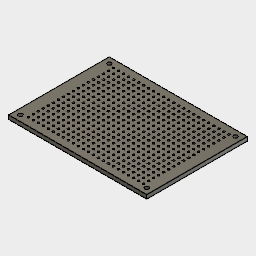
Perfboard (Autodesk Fusion 360 design; units mm, degrees)
Autodesk Fusion 360 part; units mm, degrees
sketch "Sketch3" plane through (0, 0, 0) normal (0, 1, 0) x (1, 0, 0)
  line L0 (0, 0) -> (70, 0)
  line L1 (70, 0) -> (70, 51)
  line L2 (70, 51) -> (0, 51)
  line L3 (0, 51) -> (0, 0)
  line L4 (4.5004, 2.9992) -> (65.5004, 2.9992)
  line L5 (65.5004, 2.9992) -> (65.5004, 47.9992)
  line L6 (65.5004, 47.9992) -> (4.5004, 47.9992)
  line L7 (4.5004, 47.9992) -> (4.5004, 2.9992)
  circle A0 centre (3, 3) radius 1
  circle A1 centre (3, 47.995) radius 1
  circle A2 centre (67, 3) radius 1
  circle A3 centre (67, 48) radius 1
  circle A4 centre (6, 4) radius 0.5
  circle A5 centre (6, 6.54) radius 0.5
  circle A6 centre (6, 9.08) radius 0.5
  circle A7 centre (6, 11.62) radius 0.5
  circle A8 centre (6, 21.78) radius 0.5
  circle A9 centre (6, 19.24) radius 0.5
  circle A10 centre (6, 16.7) radius 0.5
  circle A11 centre (6, 14.16) radius 0.5
  circle A12 centre (6, 24.32) radius 0.5
  circle A13 centre (6, 37.02) radius 0.5
  circle A14 centre (6, 26.86) radius 0.5
  circle A15 centre (6, 39.56) radius 0.5
  circle A16 centre (6, 29.4) radius 0.5
  circle A17 centre (6, 42.1) radius 0.5
  circle A18 centre (6, 34.48) radius 0.5
  circle A19 centre (6, 31.94) radius 0.5
  circle A20 centre (6, 44.64) radius 0.5
  circle A21 centre (6, 47.18) radius 0.5
  circle A22 centre (8.54, 6.54) radius 0.5
  circle A23 centre (8.54, 14.16) radius 0.5
  circle A24 centre (8.54, 24.32) radius 0.5
  circle A25 centre (8.54, 31.94) radius 0.5
  circle A26 centre (8.54, 26.86) radius 0.5
  circle A27 centre (8.54, 42.1) radius 0.5
  circle A28 centre (8.54, 34.48) radius 0.5
  circle A29 centre (8.54, 29.4) radius 0.5
  circle A30 centre (8.54, 16.7) radius 0.5
  circle A31 centre (8.54, 37.02) radius 0.5
  circle A32 centre (8.54, 21.78) radius 0.5
  circle A33 centre (8.54, 44.64) radius 0.5
  circle A34 centre (8.54, 19.24) radius 0.5
  circle A35 centre (8.54, 11.62) radius 0.5
  circle A36 centre (8.54, 4) radius 0.5
  circle A37 centre (8.54, 9.08) radius 0.5
  circle A38 centre (8.54, 39.56) radius 0.5
  circle A39 centre (8.54, 47.18) radius 0.5
  circle A40 centre (11.08, 34.48) radius 0.5
  circle A41 centre (13.62, 31.94) radius 0.5
  circle A42 centre (13.62, 19.24) radius 0.5
  circle A43 centre (11.08, 6.54) radius 0.5
  circle A44 centre (11.08, 21.78) radius 0.5
  circle A45 centre (11.08, 16.7) radius 0.5
  circle A46 centre (11.08, 14.16) radius 0.5
  circle A47 centre (11.08, 24.32) radius 0.5
  circle A48 centre (13.62, 44.64) radius 0.5
  circle A49 centre (13.62, 37.02) radius 0.5
  circle A50 centre (13.62, 16.7) radius 0.5
  circle A51 centre (13.62, 29.4) radius 0.5
  circle A52 centre (11.08, 9.08) radius 0.5
  circle A53 centre (11.08, 42.1) radius 0.5
  circle A54 centre (11.08, 26.86) radius 0.5
  circle A55 centre (13.62, 11.62) radius 0.5
  circle A56 centre (13.62, 34.48) radius 0.5
  circle A57 centre (13.62, 26.86) radius 0.5
  circle A58 centre (13.62, 6.54) radius 0.5
  circle A59 centre (13.62, 24.32) radius 0.5
  circle A60 centre (11.08, 47.18) radius 0.5
  circle A61 centre (13.62, 21.78) radius 0.5
  circle A62 centre (13.62, 42.1) radius 0.5
  circle A63 centre (11.08, 19.24) radius 0.5
  circle A64 centre (11.08, 31.94) radius 0.5
  circle A65 centre (11.08, 44.64) radius 0.5
  circle A66 centre (11.08, 4) radius 0.5
  circle A67 centre (11.08, 11.62) radius 0.5
  circle A68 centre (11.08, 37.02) radius 0.5
  circle A69 centre (11.08, 39.56) radius 0.5
  circle A70 centre (11.08, 29.4) radius 0.5
  circle A71 centre (13.62, 14.16) radius 0.5
  circle A72 centre (13.62, 39.56) radius 0.5
  circle A73 centre (13.62, 9.08) radius 0.5
  circle A74 centre (13.62, 47.18) radius 0.5
  circle A75 centre (13.62, 4) radius 0.5
  circle A76 centre (21.24, 24.32) radius 0.5
  circle A77 centre (21.24, 14.16) radius 0.5
  circle A78 centre (23.78, 6.54) radius 0.5
  circle A79 centre (21.24, 42.1) radius 0.5
  circle A80 centre (23.78, 44.64) radius 0.5
  circle A81 centre (18.7, 47.18) radius 0.5
  circle A82 centre (23.78, 34.48) radius 0.5
  circle A83 centre (23.78, 29.4) radius 0.5
  circle A84 centre (23.78, 16.7) radius 0.5
  circle A85 centre (23.78, 24.32) radius 0.5
  circle A86 centre (23.78, 26.86) radius 0.5
  circle A87 centre (21.24, 26.86) radius 0.5
  circle A88 centre (23.78, 11.62) radius 0.5
  circle A89 centre (21.24, 9.08) radius 0.5
  circle A90 centre (23.78, 37.02) radius 0.5
  circle A91 centre (23.78, 19.24) radius 0.5
  circle A92 centre (23.78, 31.94) radius 0.5
  circle A93 centre (18.7, 34.48) radius 0.5
  circle A94 centre (21.24, 34.48) radius 0.5
  circle A95 centre (16.16, 14.16) radius 0.5
  circle A96 centre (16.16, 44.64) radius 0.5
  circle A97 centre (16.16, 47.18) radius 0.5
  circle A98 centre (16.16, 34.48) radius 0.5
  circle A99 centre (16.16, 26.86) radius 0.5
  circle A100 centre (16.16, 9.08) radius 0.5
  circle A101 centre (16.16, 39.56) radius 0.5
  circle A102 centre (16.16, 31.94) radius 0.5
  circle A103 centre (16.16, 16.7) radius 0.5
  circle A104 centre (16.16, 11.62) radius 0.5
  circle A105 centre (16.16, 37.02) radius 0.5
  circle A106 centre (16.16, 19.24) radius 0.5
  circle A107 centre (16.16, 29.4) radius 0.5
  circle A108 centre (18.7, 6.54) radius 0.5
  circle A109 centre (18.7, 14.16) radius 0.5
  circle A110 centre (18.7, 24.32) radius 0.5
  circle A111 centre (16.16, 4) radius 0.5
  circle A112 centre (16.16, 21.78) radius 0.5
  circle A113 centre (18.7, 31.94) radius 0.5
  circle A114 centre (16.16, 24.32) radius 0.5
  circle A115 centre (18.7, 26.86) radius 0.5
  circle A116 centre (16.16, 42.1) radius 0.5
  circle A117 centre (18.7, 42.1) radius 0.5
  circle A118 centre (16.16, 6.54) radius 0.5
  circle A119 centre (21.24, 6.54) radius 0.5
  circle A120 centre (21.24, 16.7) radius 0.5
  circle A121 centre (18.7, 9.08) radius 0.5
  circle A122 centre (21.24, 21.78) radius 0.5
  circle A123 centre (18.7, 11.62) radius 0.5
  circle A124 centre (23.78, 39.56) radius 0.5
  circle A125 centre (21.24, 44.64) radius 0.5
  circle A126 centre (21.24, 31.94) radius 0.5
  circle A127 centre (21.24, 11.62) radius 0.5
  circle A128 centre (18.7, 37.02) radius 0.5
  circle A129 centre (21.24, 39.56) radius 0.5
  circle A130 centre (23.78, 42.1) radius 0.5
  circle A131 centre (18.7, 21.78) radius 0.5
  circle A132 centre (23.78, 21.78) radius 0.5
  circle A133 centre (23.78, 9.08) radius 0.5
  circle A134 centre (23.78, 14.16) radius 0.5
  circle A135 centre (21.24, 47.18) radius 0.5
  circle A136 centre (21.24, 19.24) radius 0.5
  circle A137 centre (18.7, 4) radius 0.5
  circle A138 centre (21.24, 4) radius 0.5
  circle A139 centre (18.7, 29.4) radius 0.5
  circle A140 centre (18.7, 44.64) radius 0.5
  circle A141 centre (21.24, 37.02) radius 0.5
  circle A142 centre (18.7, 16.7) radius 0.5
  circle A143 centre (23.78, 4) radius 0.5
  circle A144 centre (18.7, 19.24) radius 0.5
  circle A145 centre (21.24, 29.4) radius 0.5
  circle A146 centre (23.78, 47.18) radius 0.5
  circle A147 centre (18.7, 39.56) radius 0.5
  circle A148 centre (39.02, 42.1) radius 0.5
  circle A149 centre (36.48, 37.02) radius 0.5
  circle A150 centre (36.48, 11.62) radius 0.5
  circle A151 centre (41.56, 34.48) radius 0.5
  circle A152 centre (39.02, 6.54) radius 0.5
  circle A153 centre (36.48, 42.1) radius 0.5
  circle A154 centre (36.48, 19.24) radius 0.5
  circle A155 centre (36.48, 4) radius 0.5
  circle A156 centre (39.02, 26.86) radius 0.5
  circle A157 centre (36.48, 24.32) radius 0.5
  circle A158 centre (36.48, 29.4) radius 0.5
  circle A159 centre (39.02, 31.94) radius 0.5
  circle A160 centre (36.48, 21.78) radius 0.5
  circle A161 centre (39.02, 24.32) radius 0.5
  circle A162 centre (39.02, 14.16) radius 0.5
  circle A163 centre (36.48, 39.56) radius 0.5
  circle A164 centre (36.48, 9.08) radius 0.5
  circle A165 centre (31.4, 47.18) radius 0.5
  circle A166 centre (33.94, 6.54) radius 0.5
  circle A167 centre (33.94, 42.1) radius 0.5
  circle A168 centre (31.4, 31.94) radius 0.5
  circle A169 centre (31.4, 37.02) radius 0.5
  circle A170 centre (31.4, 39.56) radius 0.5
  circle A171 centre (33.94, 9.08) radius 0.5
  circle A172 centre (33.94, 47.18) radius 0.5
  circle A173 centre (33.94, 34.48) radius 0.5
  circle A174 centre (33.94, 14.16) radius 0.5
  circle A175 centre (33.94, 4) radius 0.5
  circle A176 centre (39.02, 39.56) radius 0.5
  circle A177 centre (44.1, 47.18) radius 0.5
  circle A178 centre (41.56, 29.4) radius 0.5
  circle A179 centre (33.94, 21.78) radius 0.5
  circle A180 centre (44.1, 4) radius 0.5
  circle A181 centre (39.02, 19.24) radius 0.5
  circle A182 centre (33.94, 39.56) radius 0.5
  circle A183 centre (39.02, 16.7) radius 0.5
  circle A184 centre (33.94, 24.32) radius 0.5
  circle A185 centre (41.56, 37.02) radius 0.5
  circle A186 centre (39.02, 34.48) radius 0.5
  circle A187 centre (31.4, 19.24) radius 0.5
  circle A188 centre (31.4, 29.4) radius 0.5
  circle A189 centre (33.94, 26.86) radius 0.5
  circle A190 centre (31.4, 4) radius 0.5
  circle A191 centre (31.4, 11.62) radius 0.5
  circle A192 centre (31.4, 44.64) radius 0.5
  circle A193 centre (36.48, 14.16) radius 0.5
  circle A194 centre (36.48, 16.7) radius 0.5
  circle A195 centre (36.48, 47.18) radius 0.5
  circle A196 centre (36.48, 31.94) radius 0.5
  circle A197 centre (28.86, 34.48) radius 0.5
  circle A198 centre (28.86, 42.1) radius 0.5
  circle A199 centre (31.4, 42.1) radius 0.5
  circle A200 centre (31.4, 26.86) radius 0.5
  circle A201 centre (28.86, 47.18) radius 0.5
  circle A202 centre (28.86, 37.02) radius 0.5
  circle A203 centre (28.86, 44.64) radius 0.5
  circle A204 centre (33.94, 31.94) radius 0.5
  circle A205 centre (33.94, 16.7) radius 0.5
  circle A206 centre (33.94, 11.62) radius 0.5
  circle A207 centre (31.4, 14.16) radius 0.5
  circle A208 centre (28.86, 39.56) radius 0.5
  circle A209 centre (28.86, 9.08) radius 0.5
  circle A210 centre (28.86, 4) radius 0.5
  circle A211 centre (31.4, 6.54) radius 0.5
  circle A212 centre (33.94, 37.02) radius 0.5
  circle A213 centre (28.86, 21.78) radius 0.5
  circle A214 centre (33.94, 29.4) radius 0.5
  circle A215 centre (28.86, 11.62) radius 0.5
  circle A216 centre (31.4, 34.48) radius 0.5
  circle A217 centre (28.86, 29.4) radius 0.5
  circle A218 centre (31.4, 16.7) radius 0.5
  circle A219 centre (31.4, 24.32) radius 0.5
  circle A220 centre (28.86, 16.7) radius 0.5
  circle A221 centre (33.94, 44.64) radius 0.5
  circle A222 centre (31.4, 9.08) radius 0.5
  circle A223 centre (28.86, 19.24) radius 0.5
  circle A224 centre (33.94, 19.24) radius 0.5
  circle A225 centre (31.4, 21.78) radius 0.5
  circle A226 centre (36.48, 44.64) radius 0.5
  circle A227 centre (26.32, 29.4) radius 0.5
  circle A228 centre (26.32, 4) radius 0.5
  circle A229 centre (26.32, 42.1) radius 0.5
  circle A230 centre (26.32, 21.78) radius 0.5
  circle A231 centre (26.32, 34.48) radius 0.5
  circle A232 centre (26.32, 31.94) radius 0.5
  circle A233 centre (26.32, 47.18) radius 0.5
  circle A234 centre (28.86, 6.54) radius 0.5
  circle A235 centre (26.32, 44.64) radius 0.5
  circle A236 centre (28.86, 14.16) radius 0.5
  circle A237 centre (26.32, 26.86) radius 0.5
  circle A238 centre (28.86, 24.32) radius 0.5
  circle A239 centre (26.32, 9.08) radius 0.5
  circle A240 centre (26.32, 14.16) radius 0.5
  circle A241 centre (26.32, 37.02) radius 0.5
  circle A242 centre (26.32, 39.56) radius 0.5
  circle A243 centre (26.32, 24.32) radius 0.5
  circle A244 centre (26.32, 6.54) radius 0.5
  circle A245 centre (26.32, 16.7) radius 0.5
  circle A246 centre (26.32, 11.62) radius 0.5
  circle A247 centre (26.32, 19.24) radius 0.5
  circle A248 centre (28.86, 31.94) radius 0.5
  circle A249 centre (28.86, 26.86) radius 0.5
  circle A250 centre (36.48, 26.86) radius 0.5
  circle A251 centre (41.56, 4) radius 0.5
  circle A252 centre (39.02, 4) radius 0.5
  circle A253 centre (39.02, 37.02) radius 0.5
  circle A254 centre (41.56, 44.64) radius 0.5
  circle A255 centre (44.1, 39.56) radius 0.5
  circle A256 centre (39.02, 11.62) radius 0.5
  circle A257 centre (39.02, 9.08) radius 0.5
  circle A258 centre (41.56, 6.54) radius 0.5
  circle A259 centre (36.48, 6.54) radius 0.5
  circle A260 centre (39.02, 21.78) radius 0.5
  circle A261 centre (41.56, 21.78) radius 0.5
  circle A262 centre (44.1, 14.16) radius 0.5
  circle A263 centre (41.56, 16.7) radius 0.5
  circle A264 centre (36.48, 34.48) radius 0.5
  circle A265 centre (41.56, 11.62) radius 0.5
  circle A266 centre (44.1, 9.08) radius 0.5
  circle A267 centre (39.02, 44.64) radius 0.5
  circle A268 centre (41.56, 19.24) radius 0.5
  circle A269 centre (41.56, 47.18) radius 0.5
  circle A270 centre (41.56, 39.56) radius 0.5
  circle A271 centre (44.1, 21.78) radius 0.5
  circle A272 centre (44.1, 42.1) radius 0.5
  circle A273 centre (41.56, 31.94) radius 0.5
  circle A274 centre (39.02, 29.4) radius 0.5
  circle A275 centre (44.1, 31.94) radius 0.5
  circle A276 centre (41.56, 26.86) radius 0.5
  circle A277 centre (39.02, 47.18) radius 0.5
  circle A278 centre (44.1, 19.24) radius 0.5
  circle A279 centre (41.56, 24.32) radius 0.5
  circle A280 centre (44.1, 26.86) radius 0.5
  circle A281 centre (44.1, 37.02) radius 0.5
  circle A282 centre (44.1, 44.64) radius 0.5
  circle A283 centre (44.1, 6.54) radius 0.5
  circle A284 centre (44.1, 24.32) radius 0.5
  circle A285 centre (44.1, 34.48) radius 0.5
  circle A286 centre (41.56, 14.16) radius 0.5
  circle A287 centre (41.56, 9.08) radius 0.5
  circle A288 centre (44.1, 16.7) radius 0.5
  circle A289 centre (44.1, 11.62) radius 0.5
  circle A290 centre (41.56, 42.1) radius 0.5
  circle A291 centre (44.1, 29.4) radius 0.5
  circle A292 centre (59.34, 47.18) radius 0.5
  circle A293 centre (56.8, 34.48) radius 0.5
  circle A294 centre (49.18, 29.4) radius 0.5
  circle A295 centre (49.18, 14.16) radius 0.5
  circle A296 centre (51.72, 4) radius 0.5
  circle A297 centre (54.26, 39.56) radius 0.5
  circle A298 centre (54.26, 42.1) radius 0.5
  circle A299 centre (49.18, 34.48) radius 0.5
  circle A300 centre (51.72, 21.78) radius 0.5
  circle A301 centre (46.64, 11.62) radius 0.5
  circle A302 centre (51.72, 16.7) radius 0.5
  circle A303 centre (54.26, 24.32) radius 0.5
  circle A304 centre (54.26, 14.16) radius 0.5
  circle A305 centre (46.64, 44.64) radius 0.5
  circle A306 centre (51.72, 47.18) radius 0.5
  circle A307 centre (46.64, 42.1) radius 0.5
  circle A308 centre (49.18, 44.64) radius 0.5
  circle A309 centre (46.64, 9.08) radius 0.5
  circle A310 centre (49.18, 19.24) radius 0.5
  circle A311 centre (46.64, 31.94) radius 0.5
  circle A312 centre (46.64, 39.56) radius 0.5
  circle A313 centre (49.18, 9.08) radius 0.5
  circle A314 centre (56.8, 29.4) radius 0.5
  circle A315 centre (59.34, 4) radius 0.5
  circle A316 centre (51.72, 42.1) radius 0.5
  circle A317 centre (54.26, 19.24) radius 0.5
  circle A318 centre (54.26, 16.7) radius 0.5
  circle A319 centre (49.18, 47.18) radius 0.5
  circle A320 centre (54.26, 34.48) radius 0.5
  circle A321 centre (49.18, 21.78) radius 0.5
  circle A322 centre (49.18, 31.94) radius 0.5
  circle A323 centre (51.72, 24.32) radius 0.5
  circle A324 centre (49.18, 24.32) radius 0.5
  circle A325 centre (49.18, 4) radius 0.5
  circle A326 centre (51.72, 29.4) radius 0.5
  circle A327 centre (46.64, 26.86) radius 0.5
  circle A328 centre (54.26, 6.54) radius 0.5
  circle A329 centre (51.72, 31.94) radius 0.5
  circle A330 centre (49.18, 11.62) radius 0.5
  circle A331 centre (54.26, 31.94) radius 0.5
  circle A332 centre (51.72, 14.16) radius 0.5
  circle A333 centre (46.64, 14.16) radius 0.5
  circle A334 centre (51.72, 37.02) radius 0.5
  circle A335 centre (54.26, 26.86) radius 0.5
  circle A336 centre (46.64, 19.24) radius 0.5
  circle A337 centre (51.72, 9.08) radius 0.5
  circle A338 centre (46.64, 37.02) radius 0.5
  circle A339 centre (51.72, 11.62) radius 0.5
  circle A340 centre (49.18, 39.56) radius 0.5
  circle A341 centre (49.18, 26.86) radius 0.5
  circle A342 centre (46.64, 4) radius 0.5
  circle A343 centre (46.64, 6.54) radius 0.5
  circle A344 centre (46.64, 47.18) radius 0.5
  circle A345 centre (49.18, 42.1) radius 0.5
  circle A346 centre (56.8, 37.02) radius 0.5
  circle A347 centre (49.18, 16.7) radius 0.5
  circle A348 centre (49.18, 37.02) radius 0.5
  circle A349 centre (46.64, 34.48) radius 0.5
  circle A350 centre (46.64, 16.7) radius 0.5
  circle A351 centre (49.18, 6.54) radius 0.5
  circle A352 centre (46.64, 24.32) radius 0.5
  circle A353 centre (51.72, 39.56) radius 0.5
  circle A354 centre (51.72, 19.24) radius 0.5
  circle A355 centre (46.64, 29.4) radius 0.5
  circle A356 centre (59.34, 6.54) radius 0.5
  circle A357 centre (59.34, 21.78) radius 0.5
  circle A358 centre (56.8, 31.94) radius 0.5
  circle A359 centre (56.8, 21.78) radius 0.5
  circle A360 centre (59.34, 9.08) radius 0.5
  circle A361 centre (56.8, 14.16) radius 0.5
  circle A362 centre (56.8, 4) radius 0.5
  circle A363 centre (59.34, 29.4) radius 0.5
  circle A364 centre (56.8, 47.18) radius 0.5
  circle A365 centre (56.8, 16.7) radius 0.5
  circle A366 centre (56.8, 11.62) radius 0.5
  circle A367 centre (54.26, 9.08) radius 0.5
  circle A368 centre (51.72, 26.86) radius 0.5
  circle A369 centre (59.34, 42.1) radius 0.5
  circle A370 centre (56.8, 39.56) radius 0.5
  circle A371 centre (59.34, 31.94) radius 0.5
  circle A372 centre (56.8, 6.54) radius 0.5
  circle A373 centre (56.8, 44.64) radius 0.5
  circle A374 centre (56.8, 19.24) radius 0.5
  circle A375 centre (59.34, 11.62) radius 0.5
  circle A376 centre (59.34, 39.56) radius 0.5
  circle A377 centre (59.34, 14.16) radius 0.5
  circle A378 centre (51.72, 34.48) radius 0.5
  circle A379 centre (56.8, 26.86) radius 0.5
  circle A380 centre (51.72, 6.54) radius 0.5
  circle A381 centre (54.26, 21.78) radius 0.5
  circle A382 centre (59.34, 37.02) radius 0.5
  circle A383 centre (59.34, 44.64) radius 0.5
  circle A384 centre (59.34, 24.32) radius 0.5
  circle A385 centre (54.26, 11.62) radius 0.5
  circle A386 centre (59.34, 34.48) radius 0.5
  circle A387 centre (56.8, 9.08) radius 0.5
  circle A388 centre (51.72, 44.64) radius 0.5
  circle A389 centre (54.26, 47.18) radius 0.5
  circle A390 centre (59.34, 16.7) radius 0.5
  circle A391 centre (54.26, 4) radius 0.5
  circle A392 centre (54.26, 29.4) radius 0.5
  circle A393 centre (56.8, 24.32) radius 0.5
  circle A394 centre (46.64, 21.78) radius 0.5
  circle A395 centre (56.8, 42.1) radius 0.5
  circle A396 centre (59.34, 19.24) radius 0.5
  circle A397 centre (59.34, 26.86) radius 0.5
  circle A398 centre (54.26, 44.64) radius 0.5
  circle A399 centre (54.26, 37.02) radius 0.5
  circle A400 centre (61.88, 37.02) radius 0.5
  circle A401 centre (61.88, 19.24) radius 0.5
  circle A402 centre (64.42, 47.18) radius 0.5
  circle A403 centre (64.42, 42.1) radius 0.5
  circle A404 centre (61.88, 11.62) radius 0.5
  circle A405 centre (61.88, 39.56) radius 0.5
  circle A406 centre (64.42, 39.56) radius 0.5
  circle A407 centre (61.88, 16.7) radius 0.5
  circle A408 centre (61.88, 29.4) radius 0.5
  circle A409 centre (64.42, 11.62) radius 0.5
  circle A410 centre (61.88, 34.48) radius 0.5
  circle A411 centre (61.88, 47.18) radius 0.5
  circle A412 centre (64.42, 29.4) radius 0.5
  circle A413 centre (64.42, 9.08) radius 0.5
  circle A414 centre (61.88, 14.16) radius 0.5
  circle A415 centre (61.88, 21.78) radius 0.5
  circle A416 centre (64.42, 4) radius 0.5
  circle A417 centre (64.42, 21.78) radius 0.5
  circle A418 centre (61.88, 6.54) radius 0.5
  circle A419 centre (64.42, 31.94) radius 0.5
  circle A420 centre (61.88, 44.64) radius 0.5
  circle A421 centre (61.88, 31.94) radius 0.5
  circle A422 centre (61.88, 4) radius 0.5
  circle A423 centre (64.42, 6.54) radius 0.5
  circle A424 centre (61.88, 9.08) radius 0.5
  circle A425 centre (64.42, 24.32) radius 0.5
  circle A426 centre (64.42, 44.64) radius 0.5
  circle A427 centre (64.42, 19.24) radius 0.5
  circle A428 centre (61.88, 42.1) radius 0.5
  circle A429 centre (64.42, 16.7) radius 0.5
  circle A430 centre (64.42, 34.48) radius 0.5
  circle A431 centre (61.88, 24.32) radius 0.5
  circle A432 centre (64.42, 26.86) radius 0.5
  circle A433 centre (64.42, 14.16) radius 0.5
  circle A434 centre (61.88, 26.86) radius 0.5
  circle A435 centre (64.42, 37.02) radius 0.5
  dimension "d8" = 70
  dimension "d9" = 51
  dimension "d10" = 61
  dimension "d11" = 45
  dimension "d16" = 2
  dimension "d17" = 2
  dimension "d18" = 2
  dimension "d23" = 1
  dimension "d24" = 1
  dimension "d26" = 1
  dimension "d27" = 1
  dimension "d28" = 1
  dimension "d29" = 1
  dimension "d30" = 1
  dimension "d31" = 1
  dimension "d32" = 1
  dimension "d33" = 1
  dimension "d34" = 1
  dimension "d35" = 1
  dimension "d36" = 1
  dimension "d37" = 1
  dimension "d38" = 1
  dimension "d39" = 1
  dimension "d40" = 1
  dimension "d41" = 1
  dimension "d42" = 1
  dimension "d43" = 1
  dimension "d44" = 1
  dimension "d45" = 1
  dimension "d46" = 1
  dimension "d47" = 1
  dimension "d48" = 1
  dimension "d49" = 1
  dimension "d50" = 1
  dimension "d51" = 1
  dimension "d52" = 1
  dimension "d53" = 1
  dimension "d54" = 1
  dimension "d55" = 1
  dimension "d56" = 1
  dimension "d57" = 1
  dimension "d58" = 1
  dimension "d59" = 1
  dimension "d60" = 1
  dimension "d61" = 1
  dimension "d62" = 1
  dimension "d63" = 1
  dimension "d64" = 1
  dimension "d65" = 1
  dimension "d66" = 1
  dimension "d67" = 1
  dimension "d68" = 1
  dimension "d69" = 1
  dimension "d70" = 1
  dimension "d71" = 1
  dimension "d72" = 1
  dimension "d73" = 1
  dimension "d74" = 1
  dimension "d75" = 1
  dimension "d76" = 1
  dimension "d77" = 1
  dimension "d78" = 1
  dimension "d79" = 1
  dimension "d80" = 1
  dimension "d81" = 1
  dimension "d82" = 1
  dimension "d83" = 1
  dimension "d84" = 1
  dimension "d85" = 1
  dimension "d86" = 1
  dimension "d87" = 1
  dimension "d88" = 1
  dimension "d89" = 1
  dimension "d90" = 1
  dimension "d91" = 1
  dimension "d92" = 1
  dimension "d93" = 1
  dimension "d94" = 1
  dimension "d95" = 1
  dimension "d96" = 1
  dimension "d97" = 1
  dimension "d98" = 1
  dimension "d99" = 1
  dimension "d100" = 1
  dimension "d101" = 1
  dimension "d102" = 1
  dimension "d103" = 1
  dimension "d104" = 1
  dimension "d105" = 1
  dimension "d106" = 1
  dimension "d107" = 1
  dimension "d108" = 1
  dimension "d109" = 1
  dimension "d110" = 1
  dimension "d111" = 1
  dimension "d112" = 1
  dimension "d113" = 1
  dimension "d114" = 1
  dimension "d115" = 1
  dimension "d116" = 1
  dimension "d117" = 1
  dimension "d118" = 1
  dimension "d119" = 1
  dimension "d120" = 1
  dimension "d121" = 1
  dimension "d122" = 1
  dimension "d123" = 1
  dimension "d124" = 1
  dimension "d125" = 1
  dimension "d126" = 1
  dimension "d127" = 1
  dimension "d128" = 1
  dimension "d129" = 1
  dimension "d130" = 1
  dimension "d131" = 1
  dimension "d132" = 1
  dimension "d133" = 1
  dimension "d134" = 1
  dimension "d135" = 1
  dimension "d136" = 1
  dimension "d137" = 1
  dimension "d138" = 1
  dimension "d139" = 1
  dimension "d140" = 1
  dimension "d141" = 1
  dimension "d142" = 1
  dimension "d143" = 1
  dimension "d144" = 1
  dimension "d145" = 1
  dimension "d146" = 1
  dimension "d147" = 1
  dimension "d148" = 1
  dimension "d149" = 1
  dimension "d150" = 1
  dimension "d151" = 1
  dimension "d152" = 1
  dimension "d153" = 1
  dimension "d154" = 1
  dimension "d155" = 1
  dimension "d156" = 1
  dimension "d157" = 1
  dimension "d158" = 1
  dimension "d159" = 1
  dimension "d160" = 1
  dimension "d161" = 1
  dimension "d162" = 1
  dimension "d163" = 1
  dimension "d164" = 1
  dimension "d165" = 1
  dimension "d166" = 1
  dimension "d167" = 1
  dimension "d168" = 1
  dimension "d169" = 1
  dimension "d170" = 1
  dimension "d171" = 1
  dimension "d172" = 1
  dimension "d173" = 1
  dimension "d174" = 1
  dimension "d175" = 1
  dimension "d176" = 1
  dimension "d177" = 1
  dimension "d178" = 1
  dimension "d179" = 1
  dimension "d180" = 1
  dimension "d181" = 1
  dimension "d182" = 1
  dimension "d183" = 1
  dimension "d184" = 1
  dimension "d185" = 1
  dimension "d186" = 1
  dimension "d187" = 1
  dimension "d188" = 1
  dimension "d189" = 1
  dimension "d190" = 1
  dimension "d191" = 1
  dimension "d192" = 1
  dimension "d193" = 1
  dimension "d194" = 1
  dimension "d195" = 1
  dimension "d196" = 1
  dimension "d197" = 1
  dimension "d198" = 1
  dimension "d199" = 1
  dimension "d200" = 1
  dimension "d201" = 1
  dimension "d202" = 1
  dimension "d203" = 1
  dimension "d204" = 1
  dimension "d205" = 1
  dimension "d206" = 1
  dimension "d207" = 1
  dimension "d208" = 1
  dimension "d209" = 1
  dimension "d210" = 1
  dimension "d211" = 1
  dimension "d212" = 1
  dimension "d213" = 1
  dimension "d214" = 1
  dimension "d215" = 1
  dimension "d216" = 1
  dimension "d217" = 1
  dimension "d218" = 1
  dimension "d219" = 1
  dimension "d220" = 1
  dimension "d221" = 1
  dimension "d222" = 1
  dimension "d223" = 1
  dimension "d224" = 1
  dimension "d225" = 1
  dimension "d226" = 1
  dimension "d227" = 1
  dimension "d228" = 1
  dimension "d229" = 1
  dimension "d230" = 1
  dimension "d231" = 1
  dimension "d232" = 1
  dimension "d233" = 1
  dimension "d234" = 1
  dimension "d235" = 1
  dimension "d236" = 1
  dimension "d237" = 1
  dimension "d238" = 1
  dimension "d239" = 1
  dimension "d240" = 1
  dimension "d241" = 1
  dimension "d242" = 1
  dimension "d243" = 1
  dimension "d244" = 1
  dimension "d245" = 1
  dimension "d246" = 1
  dimension "d247" = 1
  dimension "d248" = 1
  dimension "d249" = 1
  dimension "d250" = 1
  dimension "d251" = 1
  dimension "d252" = 1
  dimension "d253" = 1
  dimension "d254" = 1
  dimension "d255" = 1
  dimension "d256" = 1
  dimension "d257" = 1
  dimension "d258" = 1
  dimension "d259" = 1
  dimension "d260" = 1
  dimension "d261" = 1
  dimension "d262" = 1
  dimension "d263" = 1
  dimension "d264" = 1
  dimension "d265" = 1
  dimension "d266" = 1
  dimension "d267" = 1
  dimension "d268" = 1
  dimension "d269" = 1
  dimension "d270" = 1
  dimension "d271" = 1
  dimension "d272" = 1
  dimension "d273" = 1
  dimension "d274" = 1
  dimension "d275" = 1
  dimension "d276" = 1
  dimension "d277" = 1
  dimension "d278" = 1
  dimension "d279" = 1
  dimension "d280" = 1
  dimension "d281" = 1
  dimension "d282" = 1
  dimension "d283" = 1
  dimension "d284" = 1
  dimension "d285" = 1
  dimension "d286" = 1
  dimension "d287" = 1
  dimension "d288" = 1
  dimension "d289" = 1
  dimension "d290" = 1
  dimension "d291" = 1
  dimension "d292" = 1
  dimension "d293" = 1
  dimension "d294" = 1
  dimension "d295" = 1
  dimension "d296" = 1
  dimension "d297" = 1
  dimension "d298" = 1
  dimension "d299" = 1
  dimension "d300" = 1
  dimension "d301" = 1
  dimension "d302" = 1
  dimension "d303" = 1
  dimension "d304" = 1
  dimension "d305" = 1
  dimension "d306" = 1
  dimension "d307" = 1
  dimension "d308" = 1
  dimension "d309" = 1
  dimension "d310" = 1
  dimension "d311" = 1
  dimension "d312" = 1
  dimension "d313" = 1
  dimension "d314" = 1
  dimension "d315" = 1
  dimension "d316" = 1
  dimension "d317" = 1
  dimension "d318" = 1
  dimension "d319" = 1
  dimension "d320" = 1
  dimension "d321" = 1
  dimension "d322" = 1
  dimension "d323" = 1
  dimension "d324" = 1
  dimension "d325" = 1
  dimension "d326" = 1
  dimension "d327" = 1
  dimension "d328" = 1
  dimension "d329" = 1
  dimension "d330" = 1
  dimension "d331" = 1
  dimension "d332" = 1
  dimension "d333" = 1
  dimension "d334" = 1
  dimension "d335" = 1
  dimension "d336" = 1
  dimension "d337" = 1
  dimension "d338" = 1
  dimension "d339" = 1
  dimension "d340" = 1
  dimension "d341" = 1
  dimension "d342" = 1
  dimension "d343" = 1
  dimension "d344" = 1
  dimension "d345" = 1
  dimension "d346" = 1
  dimension "d347" = 1
  dimension "d348" = 1
  dimension "d349" = 1
  dimension "d350" = 1
  dimension "d351" = 1
  dimension "d352" = 1
  dimension "d353" = 1
  dimension "d354" = 1
  dimension "d355" = 1
  dimension "d356" = 1
  dimension "d357" = 1
  dimension "d358" = 1
  dimension "d359" = 1
  dimension "d360" = 1
  dimension "d361" = 1
  dimension "d362" = 1
  dimension "d363" = 1
  dimension "d364" = 1
  dimension "d365" = 1
  dimension "d366" = 1
  dimension "d367" = 1
  dimension "d368" = 1
  dimension "d369" = 1
  dimension "d370" = 1
  dimension "d371" = 1
  dimension "d372" = 1
  dimension "d373" = 1
  dimension "d374" = 1
  dimension "d375" = 1
  dimension "d376" = 1
  dimension "d377" = 1
  dimension "d378" = 1
  dimension "d379" = 1
  dimension "d380" = 1
  dimension "d381" = 1
  dimension "d382" = 1
  dimension "d383" = 1
  dimension "d384" = 1
  dimension "d385" = 1
  dimension "d386" = 1
  dimension "d387" = 1
  dimension "d388" = 1
  dimension "d389" = 1
  dimension "d390" = 1
  dimension "d391" = 1
  dimension "d392" = 1
  dimension "d393" = 1
  dimension "d394" = 1
  dimension "d395" = 1
  dimension "d396" = 1
  dimension "d397" = 1
  dimension "d398" = 1
  dimension "d399" = 1
  dimension "d400" = 1
  dimension "d401" = 1
  dimension "d402" = 1
  dimension "d403" = 1
  dimension "d404" = 1
  dimension "d405" = 1
  dimension "d406" = 1
  dimension "d407" = 1
  dimension "d408" = 1
  dimension "d409" = 1
  dimension "d410" = 1
  dimension "d411" = 1
  dimension "d412" = 1
  dimension "d413" = 1
  dimension "d414" = 1
  dimension "d415" = 1
  dimension "d416" = 1
  dimension "d417" = 1
  dimension "d418" = 1
  dimension "d419" = 1
  dimension "d420" = 1
  dimension "d421" = 1
  dimension "d422" = 1
  dimension "d423" = 1
  dimension "d424" = 1
  dimension "d425" = 1
  dimension "d426" = 1
  dimension "d427" = 1
  dimension "d428" = 1
  dimension "d429" = 1
  dimension "d430" = 1
  dimension "d431" = 1
  dimension "d432" = 1
  dimension "d433" = 1
  dimension "d434" = 1
  dimension "d435" = 1
  dimension "d436" = 1
  dimension "d437" = 1
  dimension "d438" = 1
  dimension "d439" = 1
  dimension "d440" = 1
  dimension "d441" = 1
  dimension "d442" = 1
  dimension "d443" = 1
  dimension "d444" = 1
  dimension "d445" = 1
  dimension "d446" = 1
  dimension "d447" = 1
  dimension "d448" = 1
  dimension "d449" = 1
  dimension "d450" = 1
  dimension "d451" = 1
  dimension "d452" = 1
  dimension "d453" = 1
  dimension "d454" = 1
  dimension "d455" = 1
  constraint horizontal L0
  constraint vertical L1
  constraint horizontal L2
  constraint vertical L3
  constraint horizontal L4
  constraint vertical L5
  constraint horizontal L6
  constraint vertical L7
  measures "d16" diameter of A1
  measures "d17" diameter of A2
  measures "d18" diameter of A3
  measures "d23" diameter of A4
  measures "d24" diameter of A5
  measures "d26" diameter of A6
  measures "d27" diameter of A7
  measures "d28" diameter of A11
  measures "d29" diameter of A10
  measures "d30" diameter of A9
  measures "d31" diameter of A8
  measures "d32" diameter of A12
  measures "d33" diameter of A14
  measures "d34" diameter of A16
  measures "d35" diameter of A19
  measures "d36" diameter of A18
  measures "d37" diameter of A13
  measures "d38" diameter of A15
  measures "d39" diameter of A17
  measures "d40" diameter of A20
  measures "d41" diameter of A21
  measures "d42" diameter of A22
  measures "d43" diameter of A35
  measures "d44" diameter of A23
  measures "d45" diameter of A30
  measures "d46" diameter of A34
  measures "d47" diameter of A32
  measures "d48" diameter of A24
  measures "d49" diameter of A26
  measures "d50" diameter of A29
  measures "d51" diameter of A25
  measures "d52" diameter of A28
  measures "d53" diameter of A31
  measures "d54" diameter of A27
  measures "d55" diameter of A33
  measures "d56" diameter of A36
  measures "d57" diameter of A37
  measures "d58" diameter of A38
  measures "d59" diameter of A39
  measures "d60" diameter of A66
  measures "d61" diameter of A43
  measures "d62" diameter of A52
  measures "d63" diameter of A67
  measures "d64" diameter of A46
  measures "d65" diameter of A45
  measures "d66" diameter of A63
  measures "d67" diameter of A44
  measures "d68" diameter of A47
  measures "d69" diameter of A54
  measures "d70" diameter of A70
  measures "d71" diameter of A64
  measures "d72" diameter of A40
  measures "d73" diameter of A68
  measures "d74" diameter of A69
  measures "d75" diameter of A53
  measures "d76" diameter of A65
  measures "d77" diameter of A60
  measures "d78" diameter of A58
  measures "d79" diameter of A55
  measures "d80" diameter of A71
  measures "d81" diameter of A50
  measures "d82" diameter of A42
  measures "d83" diameter of A61
  measures "d84" diameter of A59
  measures "d85" diameter of A57
  measures "d86" diameter of A51
  measures "d87" diameter of A41
  measures "d88" diameter of A56
  measures "d89" diameter of A49
  measures "d90" diameter of A62
  measures "d91" diameter of A48
  measures "d92" diameter of A75
  measures "d93" diameter of A73
  measures "d94" diameter of A72
  measures "d95" diameter of A74
  measures "d96" diameter of A111
  measures "d97" diameter of A118
  measures "d98" diameter of A100
  measures "d99" diameter of A104
  measures "d100" diameter of A95
  measures "d101" diameter of A103
  measures "d102" diameter of A106
  measures "d103" diameter of A112
  measures "d104" diameter of A114
  measures "d105" diameter of A99
  measures "d106" diameter of A107
  measures "d107" diameter of A102
  measures "d108" diameter of A98
  measures "d109" diameter of A105
  measures "d110" diameter of A101
  measures "d111" diameter of A116
  measures "d112" diameter of A96
  measures "d113" diameter of A97
  measures "d114" diameter of A108
  measures "d115" diameter of A123
  measures "d116" diameter of A109
  measures "d117" diameter of A142
  measures "d118" diameter of A144
  measures "d119" diameter of A131
  measures "d120" diameter of A110
  measures "d121" diameter of A115
  measures "d122" diameter of A139
  measures "d123" diameter of A113
  measures "d124" diameter of A93
  measures "d125" diameter of A128
  measures "d126" diameter of A117
  measures "d127" diameter of A140
  measures "d128" diameter of A137
  measures "d129" diameter of A121
  measures "d130" diameter of A147
  measures "d131" diameter of A81
  measures "d132" diameter of A138
  measures "d133" diameter of A119
  measures "d134" diameter of A89
  measures "d135" diameter of A127
  measures "d136" diameter of A77
  measures "d137" diameter of A120
  measures "d138" diameter of A136
  measures "d139" diameter of A122
  measures "d140" diameter of A76
  measures "d141" diameter of A87
  measures "d142" diameter of A145
  measures "d143" diameter of A126
  measures "d144" diameter of A94
  measures "d145" diameter of A141
  measures "d146" diameter of A129
  measures "d147" diameter of A79
  measures "d148" diameter of A125
  measures "d149" diameter of A135
  measures "d150" diameter of A78
  measures "d151" diameter of A88
  measures "d152" diameter of A134
  measures "d153" diameter of A84
  measures "d154" diameter of A91
  measures "d155" diameter of A132
  measures "d156" diameter of A85
  measures "d157" diameter of A86
  measures "d158" diameter of A83
  measures "d159" diameter of A92
  measures "d160" diameter of A82
  measures "d161" diameter of A90
  measures "d162" diameter of A130
  measures "d163" diameter of A80
  measures "d164" diameter of A143
  measures "d165" diameter of A133
  measures "d166" diameter of A124
  measures "d167" diameter of A146
  measures "d168" diameter of A228
  measures "d169" diameter of A244
  measures "d170" diameter of A239
  measures "d171" diameter of A246
  measures "d172" diameter of A240
  measures "d173" diameter of A245
  measures "d174" diameter of A247
  measures "d175" diameter of A230
  measures "d176" diameter of A243
  measures "d177" diameter of A237
  measures "d178" diameter of A227
  measures "d179" diameter of A232
  measures "d180" diameter of A231
  measures "d181" diameter of A241
  measures "d182" diameter of A242
  measures "d183" diameter of A229
  measures "d184" diameter of A235
  measures "d185" diameter of A233
  measures "d186" diameter of A234
  measures "d187" diameter of A215
  measures "d188" diameter of A236
  measures "d189" diameter of A220
  measures "d190" diameter of A223
  measures "d191" diameter of A213
  measures "d192" diameter of A238
  measures "d193" diameter of A249
  measures "d194" diameter of A217
  measures "d195" diameter of A248
  measures "d196" diameter of A197
  measures "d197" diameter of A202
  measures "d198" diameter of A198
  measures "d199" diameter of A203
  measures "d200" diameter of A210
  measures "d201" diameter of A209
  measures "d202" diameter of A208
  measures "d203" diameter of A201
  measures "d204" diameter of A190
  measures "d205" diameter of A211
  measures "d206" diameter of A222
  measures "d207" diameter of A191
  measures "d208" diameter of A207
  measures "d209" diameter of A218
  measures "d210" diameter of A187
  measures "d211" diameter of A225
  measures "d212" diameter of A219
  measures "d213" diameter of A200
  measures "d214" diameter of A188
  measures "d215" diameter of A168
  measures "d216" diameter of A216
  measures "d217" diameter of A169
  measures "d218" diameter of A170
  measures "d219" diameter of A199
  measures "d220" diameter of A192
  measures "d221" diameter of A165
  measures "d222" diameter of A166
  measures "d223" diameter of A206
  measures "d224" diameter of A174
  measures "d225" diameter of A205
  measures "d226" diameter of A224
  measures "d227" diameter of A179
  measures "d228" diameter of A184
  measures "d229" diameter of A189
  measures "d230" diameter of A214
  measures "d231" diameter of A204
  measures "d232" diameter of A173
  measures "d233" diameter of A212
  measures "d234" diameter of A167
  measures "d235" diameter of A221
  measures "d236" diameter of A175
  measures "d237" diameter of A171
  measures "d238" diameter of A182
  measures "d239" diameter of A172
  measures "d240" diameter of A155
  measures "d241" diameter of A259
  measures "d242" diameter of A164
  measures "d243" diameter of A150
  measures "d244" diameter of A193
  measures "d245" diameter of A194
  measures "d246" diameter of A154
  measures "d247" diameter of A160
  measures "d248" diameter of A157
  measures "d249" diameter of A250
  measures "d250" diameter of A158
  measures "d251" diameter of A196
  measures "d252" diameter of A264
  measures "d253" diameter of A149
  measures "d254" diameter of A163
  measures "d255" diameter of A153
  measures "d256" diameter of A226
  measures "d257" diameter of A195
  measures "d258" diameter of A152
  measures "d259" diameter of A256
  measures "d260" diameter of A162
  measures "d261" diameter of A183
  measures "d262" diameter of A181
  measures "d263" diameter of A260
  measures "d264" diameter of A161
  measures "d265" diameter of A156
  measures "d266" diameter of A274
  measures "d267" diameter of A159
  measures "d268" diameter of A186
  measures "d269" diameter of A253
  measures "d270" diameter of A148
  measures "d271" diameter of A267
  measures "d272" diameter of A252
  measures "d273" diameter of A257
  measures "d274" diameter of A176
  measures "d275" diameter of A277
  measures "d276" diameter of A251
  measures "d277" diameter of A258
  measures "d278" diameter of A287
  measures "d279" diameter of A265
  measures "d280" diameter of A286
  measures "d281" diameter of A263
  measures "d282" diameter of A268
  measures "d283" diameter of A261
  measures "d284" diameter of A279
  measures "d285" diameter of A276
  measures "d286" diameter of A178
  measures "d287" diameter of A273
  measures "d288" diameter of A151
  measures "d289" diameter of A185
  measures "d290" diameter of A270
  measures "d291" diameter of A290
  measures "d292" diameter of A254
  measures "d293" diameter of A269
  measures "d294" diameter of A283
  measures "d295" diameter of A289
  measures "d296" diameter of A262
  measures "d297" diameter of A288
  measures "d298" diameter of A278
  measures "d299" diameter of A271
  measures "d300" diameter of A284
  measures "d301" diameter of A280
  measures "d302" diameter of A291
  measures "d303" diameter of A275
  measures "d304" diameter of A285
  measures "d305" diameter of A281
  measures "d306" diameter of A272
  measures "d307" diameter of A282
  measures "d308" diameter of A180
  measures "d309" diameter of A266
  measures "d310" diameter of A255
  measures "d311" diameter of A177
  measures "d312" diameter of A342
  measures "d313" diameter of A343
  measures "d314" diameter of A309
  measures "d315" diameter of A301
  measures "d316" diameter of A333
  measures "d317" diameter of A350
  measures "d318" diameter of A336
  measures "d319" diameter of A394
  measures "d320" diameter of A352
  measures "d321" diameter of A327
  measures "d322" diameter of A355
  measures "d323" diameter of A311
  measures "d324" diameter of A349
  measures "d325" diameter of A338
  measures "d326" diameter of A312
  measures "d327" diameter of A307
  measures "d328" diameter of A305
  measures "d329" diameter of A344
  measures "d330" diameter of A351
  measures "d331" diameter of A330
  measures "d332" diameter of A295
  measures "d333" diameter of A347
  measures "d334" diameter of A310
  measures "d335" diameter of A321
  measures "d336" diameter of A324
  measures "d337" diameter of A341
  measures "d338" diameter of A294
  measures "d339" diameter of A322
  measures "d340" diameter of A299
  measures "d341" diameter of A348
  measures "d342" diameter of A345
  measures "d343" diameter of A308
  measures "d344" diameter of A325
  measures "d345" diameter of A313
  measures "d346" diameter of A340
  measures "d347" diameter of A319
  measures "d348" diameter of A296
  measures "d349" diameter of A380
  measures "d350" diameter of A337
  measures "d351" diameter of A339
  measures "d352" diameter of A332
  measures "d353" diameter of A302
  measures "d354" diameter of A354
  measures "d355" diameter of A300
  measures "d356" diameter of A323
  measures "d357" diameter of A368
  measures "d358" diameter of A326
  measures "d359" diameter of A329
  measures "d360" diameter of A378
  measures "d361" diameter of A334
  measures "d362" diameter of A353
  measures "d363" diameter of A316
  measures "d364" diameter of A388
  measures "d365" diameter of A306
  measures "d366" diameter of A328
  measures "d367" diameter of A385
  measures "d368" diameter of A304
  measures "d369" diameter of A318
  measures "d370" diameter of A317
  measures "d371" diameter of A381
  measures "d372" diameter of A303
  measures "d373" diameter of A335
  measures "d374" diameter of A392
  measures "d375" diameter of A331
  measures "d376" diameter of A320
  measures "d377" diameter of A399
  measures "d378" diameter of A298
  measures "d379" diameter of A398
  measures "d380" diameter of A391
  measures "d381" diameter of A367
  measures "d382" diameter of A297
  measures "d383" diameter of A389
  measures "d384" diameter of A362
  measures "d385" diameter of A372
  measures "d386" diameter of A387
  measures "d387" diameter of A366
  measures "d388" diameter of A361
  measures "d389" diameter of A365
  measures "d390" diameter of A374
  measures "d391" diameter of A359
  measures "d392" diameter of A393
  measures "d393" diameter of A379
  measures "d394" diameter of A314
  measures "d395" diameter of A358
  measures "d396" diameter of A293
  measures "d397" diameter of A346
  measures "d398" diameter of A370
  measures "d399" diameter of A395
  measures "d400" diameter of A373
  measures "d401" diameter of A364
  measures "d402" diameter of A356
  measures "d403" diameter of A375
  measures "d404" diameter of A377
  measures "d405" diameter of A390
  measures "d406" diameter of A396
  measures "d407" diameter of A357
  measures "d408" diameter of A384
  measures "d409" diameter of A397
  measures "d410" diameter of A363
  measures "d411" diameter of A371
  measures "d412" diameter of A386
  measures "d413" diameter of A382
  measures "d414" diameter of A369
  measures "d415" diameter of A383
  measures "d416" diameter of A315
  measures "d417" diameter of A360
  measures "d418" diameter of A376
  measures "d419" diameter of A292
  measures "d420" diameter of A422
  measures "d421" diameter of A418
  measures "d422" diameter of A424
  measures "d423" diameter of A404
  measures "d424" diameter of A414
  measures "d425" diameter of A407
  measures "d426" diameter of A401
  measures "d427" diameter of A415
  measures "d428" diameter of A431
  measures "d429" diameter of A434
  measures "d430" diameter of A408
  measures "d431" diameter of A421
  measures "d432" diameter of A410
  measures "d433" diameter of A400
  measures "d434" diameter of A405
  measures "d435" diameter of A428
  measures "d436" diameter of A420
  measures "d437" diameter of A411
  measures "d438" diameter of A423
  measures "d439" diameter of A409
  measures "d440" diameter of A433
  measures "d441" diameter of A429
  measures "d442" diameter of A427
  measures "d443" diameter of A417
  measures "d444" diameter of A425
  measures "d445" diameter of A432
  measures "d446" diameter of A412
  measures "d447" diameter of A419
  measures "d448" diameter of A430
  measures "d449" diameter of A435
  measures "d450" diameter of A403
  measures "d451" diameter of A426
  measures "d452" diameter of A416
  measures "d453" diameter of A413
  measures "d454" diameter of A406
  measures "d455" diameter of A402
extrude "Extrude5" add sketch "Sketch3" along normal blind 2 contours L0 L1 L2 L3 | L4 L5 L6 L7
